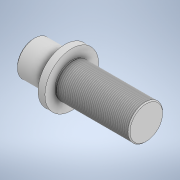
# Autodesk Inventor part: 부품3
Saved by Autodesk Inventor 2022 (Build 260153000, 153)
## iProperties
Created: 2022-09-19
Part Number: 부품3
Material: 일반
Document SubType Name: Modeling
Designer: USER
Density: 1 g/cm^3
Appearance: 기본값
Author: USER
Autodesk Inventor part; units mm, degrees
ref_plane "YZ Plane" through (0, 0, 0) normal (1, 0, 0) x (0, 1, 0)
ref_plane "XZ Plane" through (0, 0, 0) normal (0, 1, 0) x (-1, 0, 0)
ref_plane "XY Plane" through (0, 0, 0) normal (0, 0, 1) x (1, 0, 0)
sketch "스케치1" plane through (0, 0, 0) normal (0, 0, 1) x (1, 0, 0)
  line L0 (-35.0233, -0.5172) -> (35.879, -0.5172)
  line L1 (-23.7824, -0.5172) -> (-5.7824, -0.5172)
  line L2 (-5.7824, -0.5172) -> (-5.7824, 9.4828)
  line L3 (-5.7824, 9.4828) -> (-23.7824, 9.4828)
  line L4 (-23.7824, 9.4828) -> (-23.7824, -0.5172)
  line L5 (-5.7824, -0.5172) -> (-1.7824, -0.5172)
  line L6 (-1.7824, -0.5172) -> (-1.7824, 14.9828)
  line L7 (-1.7824, 14.9828) -> (-5.7824, 14.9828)
  line L8 (-5.7824, 14.9828) -> (-5.7824, -0.5172)
  line L9 (-1.7824, -0.5172) -> (41.2176, -0.5172)
  line L10 (41.2176, -0.5172) -> (41.2176, 9.4828)
  line L11 (41.2176, 9.4828) -> (-0.6628, 9.4828)
  line L12 (-1.7824, 9.4828) -> (-1.7824, -0.5172)
  line L13 (-1.7824, 9.1828) -> (-1.1824, 9.1828)
  line L14 (-1.1824, 9.1828) -> (-0.6628, 9.4828)
  point P0 (0, 0)
  point P1 (1.9905, 9.4828)
  dimension "d0" = 18
  dimension "d1" = 43
  dimension "d2" = 65
  dimension "d3" = 20
  dimension "d4" = 20
  dimension "d5" = 31
  dimension "d6" = 0.6
  dimension "d7" = 0.6
  dimension "d8" = 30
  constraints: 30 end point, 6 parallel, 4 horizontal, 4 perpendicular, 3 point on line, 1 horizontal alignment
  measures "d0" distance of L3.end L2.end
  measures "d1" distance of L10.end L12.start
  measures "d2" distance between parallel lines of L4 L10
  measures "d3" diameter of L3 L0
  measures "d4" diameter of L11 L0
  measures "d5" diameter of L7 L0
  measures "d6" distance of L13.start L13.end
  measures "d7" distance of L11.end L13.end
  measures "d8" angle of L11 L14
revolve "회전1" add sketch "스케치1" angle 360 about axis through (-35.0233, -0.5172, 0) along (1, 0, 0)
chamfer "모따기1" distance 0.6 angle 45 1 edges at (-23.7824, -10.5172, 0)
chamfer "모따기2" distance 0.6 angle 45 1 edges at (41.2176, -10.5172, 0)
thread "스레드1" size "M20x1" class "6g" standard "ISO Metric profile" full length
